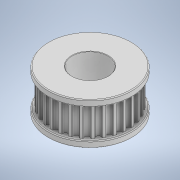
# Autodesk Inventor part: Pully_30_Rang
Saved by Autodesk Inventor 2022 (Build 260153000, 153)
## iProperties
Created: 2022-11-14
Part Number: Pully_30_Rang
Material: Generic
Document SubType Name: Modeling
Designer: nguye
Density: 1 g/cm^3
Appearance: Default
Author: nguye
Autodesk Inventor part; units mm, degrees
ref_plane "YZ Plane" through (0, 0, 0) normal (1, 0, 0) x (0, 1, 0)
ref_plane "XZ Plane" through (0, 0, 0) normal (0, 1, 0) x (-1, 0, 0)
sketch "Sketch1" plane through (0, 0, 0) normal (0, 1, 0) x (-1, 0, 0)
  circle A0 centre (0, 0) radius 9.295305
  circle A1 centre (0, 0) radius 8.545305
  line L0 (16.259061, 0) -> (-13.554366, 0)
  line L1 (0, -13.013427) -> (0, 13.013427)
  circle A2 centre (9.100305, 0) radius 0.555
  line L2 (0, 0) -> (12, -2.550679)
  circle A3 centre (8.901441, -1.89206) radius 0.555
  circle A4 centre (9.118108, -0.704775) radius 0.15
  circle A5 centre (9.065386, -1.206387) radius 0.15
  point P0 (9.214075, -1.226174)
  point P1 (9.267662, -0.716335)
  point P2 (9.11432, -0.554823)
  point P3 (8.545305, 0)
  point P4 (8.358569, -1.776669)
  point P5 (9.030504, -1.352275)
  dimension "d2" = 18.59061
  dimension "d3" = 0.75
  dimension "d4" = 1.11
  dimension "d5" = 78
  dimension "d6" = 12
  dimension "d7" = 0.3
  constraints: 6 centre point, 6 tangent, 2 end point, 2 equal radius, 2 point on line, 1 coincident
  measures "d2" diameter of A0
  measures "d3" radial gap between concentric circles of A0 A1
  measures "d4" diameter of A2
  measures "d5" angle of L2 L1
  measures "d6" horizontal distance of L2.start L2.end
  measures "d7" diameter of A4
sketch "Sketch1 outline for Extrusion1" plane through (0, 0, 0) normal (0, 1, 0) x (-1, 0, 0)
  arc A0 (9.214075, -1.226174) -> (9.267662, -0.716335) centre (0, 0) ccw
  arc A1 (9.030504, -1.352275) -> (9.214075, -1.226174) centre (9.065386, -1.206387) ccw
  arc A2 (8.358569, -1.776669) -> (9.030504, -1.352275) centre (8.901441, -1.89206) cw
  arc A3 (8.545305, 0) -> (8.358569, -1.776669) centre (0, 0) cw
  arc A4 (9.11432, -0.554823) -> (8.545305, 0) centre (9.100305, 0) cw
  arc A5 (9.267662, -0.716335) -> (9.11432, -0.554823) centre (9.118108, -0.704775) ccw
extrude "Extrusion1" add sketch "Sketch1 outline for Extrusion1" along normal blind 7
pattern_circular "Circular Pattern1" count 30 over 360 about axis through (0, -10, 0) along (0, 1, 0) of "Extrusion1"
sketch "Sketch5" plane through (0, 0, 0) normal (0, 1, 0) x (-1, 0, 0)
  circle A0 centre (0, 0) radius 8.545305
  arc A1 (7.806524, 3.475689) -> (6.913297, 5.022804) centre (0, 0) ccw
  circle A2 centre (0, 0) radius 10
  circle A3 centre (0, 0) radius 4.25
  dimension "d21" = 20
  dimension "d22" = 8.5
  constraints: 3 centre point, 3 coincident, 1 concentric
  measures "d21" diameter of A2
  measures "d22" diameter of A3
extrude "Extrusion4" add sketch "Sketch5" against normal blind 1.5 contours A0 | A2
extrude "Extrusion5" add sketch "Sketch5" along normal up to surface (7 mm away) contours A0
ref_plane "Work Plane2" through (0, 3.5, 0) normal (0, 1, 0) x (1, 0, 0)
mirror "Mirror2" about plane through (0, 3.5, 0) normal (0, 1, 0) of "Extrusion4"
fillet "Fillet1" radius 0.2 1 edges at (10, 7, 0)
fillet "Fillet2" radius 0.2 3 edges at (10, 8.5, 0) (10, 0, 0) (10, -1.5, 0)
chamfer "Chamfer1" distance 0.1 angle 45 2 edges at (4.25, 8.5, 0) (4.25, -1.5, 0)
sketch "Sketch6" plane through (0, -1.5, 0) normal (0, -1, 0) x (1, 0, 0)
  point P0 (0, 0)
  point P1 (-7, 0)
  point P2 (7, 0)
  dimension "d33" = 14
  dimension "d34" = 7
  constraints: 2 horizontal alignment
  measures "d33" distance of point (7, 0) point (-7, 0)
  measures "d34" distance of point (-7, 0) point (0, 0)
hole "Hole1" at (-7, -1.5, 0) at (7, -1.5, 0) direction (0, 1, 0) diameter 2.459 depth 8.8 thread size "M3x0.5" class "6H" standard "ISO Metric profile"
equation "\"d2\" = OD_"
equation "\"d3\" = H_"
equation "\"d4\" = BTD_"
equation "\"d7\" = PTR_"
equation "\"OD_\" = PD_ - 2 * U_"
equation "\"U_\" = 0.254"
equation "\"H_\" = 0.75"
equation "\"P_\" = 2"
equation "\"BTD_\" = 1.11"
equation "\"PTR_\" = 0.3"
equation "\"EX_\" = 7"
equation "\"SHIFT_\" = 5"
equation "\"PD_\" = 19.098609"
body "Solid1"
